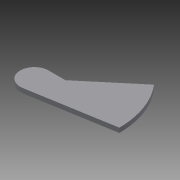
# Autodesk Inventor part: latch
Saved by Autodesk Inventor 2014 SP2 (Build 180246200, 246)
## iProperties
Created: 2015-11-29
Part Number: latch
Material: Generic
Document SubType Name: Modeling
Designer: schrluka
Density: 1 g/cm^3
Appearance: Default
Author: schrluka
Autodesk Inventor part; units mm, degrees
ref_plane "YZ Plane" through (0, 0, 0) normal (1, 0, 0) x (0, 1, 0)
ref_plane "XZ Plane" through (0, 0, 0) normal (0, 1, 0) x (-1, 0, 0)
ref_plane "XY Plane" through (0, 0, 0) normal (0, 0, 1) x (1, 0, 0)
sketch "Sketch1" plane through (0, 0, 0) normal (0, 0, 1) x (1, 0, 0)
  line L0 (0, 0) -> (75, 0) construction
  line L1 (0, 0) -> (75, 0) construction
  line L2 (0, 0) -> (57.4533, 48.2091) construction
  line L3 (0, 12.5) -> (14.8969, 12.5)
  line L4 (75, 0) -> (2.0833, -12.3252)
  arc A0 (0, 12.5) -> (2.0833, -12.3252) centre (0, 0) ccw
  arc A1 (75, 0) -> (57.4533, 48.2091) centre (0, 0) ccw
  line L5 (14.8969, 12.5) -> (57.4533, 48.2091)
  dimension "d1" = 0
  dimension "d4" = 12.5
  dimension "d7" = 12.5
  dimension "d8" = 75
  constraints: 12 end point, 4 point on circle, 3 coincident, 2 centre point, 2 collinear, 1 horizontal, 1 parallel, 1 point on line, 1 tangent
  measures "d1" distance between parallel lines of L1 L0
  measures "d4" distance from line of point (0, 0) L3
  measures "d7" radius of A0
  measures "d8" distance of L0.end point (0, 0)
extrude "Extrusion1" add sketch "Sketch1" along normal blind 4
body "Solid1"
